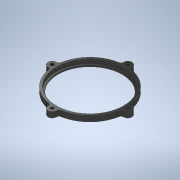
# Autodesk Inventor part: BearingClamp
Saved by Autodesk Inventor 2020 (Build 240168000, 168)
## iProperties
Created: 2019-05-28
Part Number: BearingClamp
Material: ABS Plastic
Document SubType Name: Modeling
Designer: Connor
Density: 1.06 g/cm^3
Appearance: Glossy - Black
Author: Connor
Autodesk Inventor part; units mm, degrees
ref_plane "YZ Plane" through (0, 0, 0) normal (1, 0, 0) x (0, 1, 0)
ref_plane "XZ Plane" through (0, 0, 0) normal (0, 1, 0) x (-1, 0, 0)
ref_plane "XY Plane" through (0, 0, 0) normal (0, 0, 1) x (1, 0, 0)
sketch "Sketch1" plane through (0, 0, 0) normal (0, 0, 1) x (1, 0, 0)
  line L0 (0, 0) -> (50.8, 0) construction
  line L1 (50.8, 0) -> (50.8, -6.35) construction
  line L2 (50.8, -6.35) -> (0, -6.35) construction
  line L3 (0, -6.35) -> (0, 0) construction
  line L4 (50.8, -6.35) -> (48.26, -6.35)
  line L5 (48.26, -6.35) -> (48.26, -9.525)
  line L6 (48.26, -9.525) -> (50.8, -9.525)
  line L7 (50.8, -9.525) -> (50.8, -6.35)
  line L8 (50.8, 0) -> (53.975, 0)
  line L9 (53.975, 0) -> (53.975, -9.525)
  line L10 (53.975, -9.525) -> (50.8, -9.525)
  line L11 (50.8, -9.525) -> (50.8, 0)
  dimension "d0" = 50.8
  dimension "d2" = 6.35
  dimension "d3" = 2.54
  dimension "d5" = 9.525
  dimension "d20" = 53.975
  constraints: 24 end point, 4 parallel, 4 perpendicular, 3 horizontal, 1 collinear, 1 vertical
  measures "d0" distance of L0.start L0.end
  measures "d2" distance of L2.end L0.start
  measures "d3" distance between parallel lines of L7 L5
  measures "d5" distance of L8.end L9.end
  measures "d20" distance between parallel lines of L3 L9
revolve "Revolution1" add sketch "Sketch1" angle 360 about axis through (0, -6.35, 0) along (0, 1, 0)
sketch "Sketch2" plane through (0, 0, 0) normal (0, 1, 0) x (-1, 0, 0)
  circle A0 centre (0, 0) radius 53.975 projected
  circle A1 centre (0, -57.15) radius 6.35
  circle A2 centre (0, 0) radius 53.975 projected
  circle A3 centre (9.4919, -56.3563) radius 3.175 construction
  circle A4 centre (-9.4919, -56.3563) radius 3.175 construction
  circle A5 centre (0, -57.15) radius 2.6035
  arc A6 (8.9645, -53.2253) -> (6.3279, -56.6208) centre (9.4919, -56.3563) ccw
  arc A7 (-6.3279, -56.6208) -> (-8.9645, -53.2253) centre (-9.4919, -56.3563) ccw
  point P0 (8.9645, -53.2253)
  point P1 (-8.9645, -53.2253)
  dimension "d7" = 5.207
  dimension "d16" = 57.15
  dimension "d18" = 12.7
  dimension "d19" = 6.35
  constraints: 12 point on circle, 6 centre point, 4 tangent, 3 coincident, 1 equal radius, 1 vertical alignment
  measures "d7" diameter of A5
  measures "d16" distance of point (0, 0) A1.centre
  measures "d18" diameter of A1
  measures "d19" diameter of A3
extrude "Extrusion1" add sketch "Sketch2" against normal up to surface (9.525 mm away) contours A0 A1 A7 | A6 A1 A0 | A0 A1 picked at (5.0111, -57.8774)
pattern_circular "Circular Pattern1" count 4 over 360 about axis through (0, -10, 0) along (0, 1, 0) of "Extrusion1"
fillet "Fillet1" radius 1.5875 5 edges at (-48.26, -9.525, 0) (-38.1661, -9.525, -38.1661) (-38.1661, -9.525, 38.1661) (38.1661, -9.525, 38.1661) (38.1661, -9.525, -38.1661)
body "Solid1"
